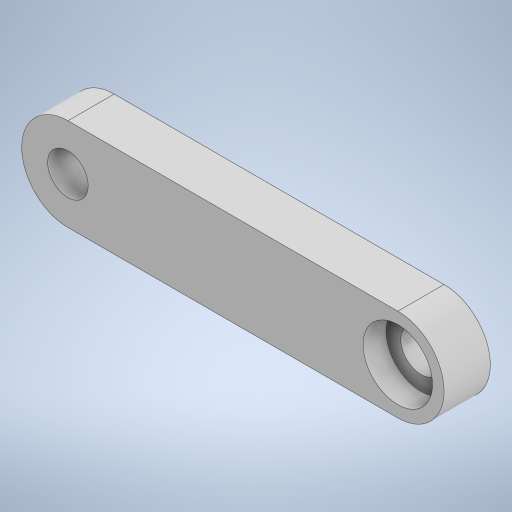
# Autodesk Inventor part: mechanism_2
Saved by Autodesk Inventor 2023 (Build 270158000, 158)
## iProperties
Created: 2024-07-18
Part Number: mechanism_2
Material: Generic
Document SubType Name: Modeling
Designer: Swoby
Density: 1 g/cm^3
Appearance: Default
Author: Swoby
Autodesk Inventor part; units mm, degrees
ref_plane "YZ Plane" through (0, 0, 0) normal (1, 0, 0) x (0, 1, 0)
ref_plane "XZ Plane" through (0, 0, 0) normal (0, 1, 0) x (-1, 0, 0)
ref_plane "XY Plane" through (0, 0, 0) normal (0, 0, 1) x (1, 0, 0)
sketch "Sketch1" plane through (0, 0, 0) normal (0, 0, 1) x (1, 0, 0)
  line L0 (-14.2785, 0) -> (14.2785, 0) construction
  line L1 (-14.2785, -4) -> (14.2785, -4)
  line L2 (14.2785, 4) -> (-14.2785, 4)
  arc A0 (-14.2785, 4) -> (-14.2785, -4) centre (-14.2785, 0) ccw
  arc A1 (14.2785, -4) -> (14.2785, 4) centre (14.2785, 0) ccw
  circle A2 centre (-14.2785, 0) radius 1.75
  circle A3 centre (14.2785, 0) radius 1.75
  point P0 (0, 0)
  dimension "d0" = 4
  dimension "d1" = 3.5
  dimension "d2" = 3.5
  dimension "d3" = 28.557
  constraints: 8 end point, 4 centre point, 4 point on circle, 4 tangent, 2 coincident, 1 horizontal, 1 midpoint, 1 parallel
  measures "d0" radius of A0
  measures "d1" diameter of A2
  measures "d2" diameter of A3
  measures "d3" distance of L0.end L0.start
extrude "Extrusion1" add sketch "Sketch1" along normal blind 4
sketch "Sketch2" plane through (0, 0, 4) normal (0, 0, 1) x (1, 0, 0)
  circle A0 centre (14.2785, 0) radius 1.75 projected
  circle A1 centre (14.2785, 0) radius 3
  point P0 (0, 0)
  dimension "d6" = 6
  constraints: 1 centre point, 1 coincident
  measures "d6" diameter of A1
extrude "Extrusion2" cut sketch "Sketch2" against normal blind 2
body "Solid1"
